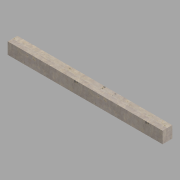
# Autodesk Inventor part: Bridge veneer
Saved by Autodesk Inventor 2022.1 (Build 261234020, 234B)
## iProperties
Created: 2021-10-21
Part Number: Bridge veneer
Material: Limestone
Document SubType Name: Modeling
Designer: awelt
Density: 2.6 g/cm^3
Appearance: Kasota Gray
Mass: 22240.5 g
Surface Area: 4243.54 cm^2
Volume: 8554.05 cm^3
Author: awelt
Autodesk Inventor part; units mm, degrees
ref_plane "YZ Plane" through (0, 0, 0) normal (1, 0, 0) x (0, 1, 0)
ref_plane "XZ Plane" through (0, 0, 0) normal (0, 1, 0) x (-1, 0, 0)
ref_plane "XY Plane" through (0, 0, 0) normal (0, 0, 1) x (1, 0, 0)
sketch "Sketch1" plane through (0, 0, 0) normal (0, 1, 0) x (-1, 0, 0)
  line L0 (609.6, -38.1) -> (-609.6, -38.1)
  line L1 (-609.6, -38.1) -> (-609.6, 38.1)
  line L2 (-609.6, 38.1) -> (609.6, 38.1)
  line L3 (609.6, 38.1) -> (609.6, -38.1)
  line L4 (609.6, -38.1) -> (-609.6, 38.1) construction
  line L5 (-609.6, -38.1) -> (609.6, 38.1) construction
  point P0 (0, 0)
  dimension "d0" = 1219.2
  dimension "d1" = 76.2
  constraints: 12 end point, 2 midpoint, 2 parallel, 1 horizontal, 1 perpendicular
  measures "d0" distance of L1.end L2.end
  measures "d1" distance of L0.end L1.end
extrude "Extrusion1" add sketch "Sketch1" along normal blind 92.075
sketch "Sketch2" plane through (609.6, 0, 38.1) normal (1, 0, 0) x (0, 0, -1)
  line L0 (0, 0) -> (0, 92.075) projected
  line L1 (0, 92.075) -> (76.2, 92.075) construction
  line L2 (0, 92.075) -> (0, 0) construction
  line L3 (0, 82.0217) -> (6.35, 82.0217)
  line L4 (6.35, 82.0217) -> (6.35, 75.6717)
  line L5 (6.35, 75.6717) -> (0, 75.6717)
  line L6 (0, 75.6717) -> (0, 82.0217) construction
  line L7 (0, 82.0217) -> (0, 75.6717)
  line L8 (0, 65.6184) -> (6.35, 65.6184)
  line L9 (6.35, 65.6184) -> (6.35, 59.2684)
  line L10 (6.35, 59.2684) -> (0, 59.2684)
  line L11 (0, 59.2684) -> (0, 65.6184)
  line L12 (0, 49.215) -> (6.35, 49.215)
  line L13 (6.35, 49.215) -> (6.35, 42.865)
  line L14 (6.35, 42.865) -> (0, 42.865)
  line L15 (0, 42.865) -> (0, 49.215)
  line L16 (0, 32.8117) -> (6.35, 32.8117)
  line L17 (6.35, 32.8117) -> (6.35, 26.4617)
  line L18 (6.35, 26.4617) -> (0, 26.4617)
  line L19 (0, 26.4617) -> (0, 32.8117)
  line L20 (0, 16.4084) -> (6.35, 16.4084)
  line L21 (6.35, 16.4084) -> (6.35, 10.0584)
  line L22 (6.35, 10.0584) -> (0, 10.0584)
  line L23 (0, 10.0584) -> (0, 16.4084)
  point P0 (38.1, 0)
  point P1 (0, 16.4084)
  point P2 (0, 10.0584)
  point P3 (0, 32.8117)
  point P4 (0, 26.4617)
  point P5 (0, 49.215)
  point P6 (0, 65.6184)
  point P7 (0, 59.2684)
  point P8 (0, 82.0217)
  point P9 (0, 75.6717)
  dimension "d5" = 6.35
  dimension "d6" = 6.35
  dimension "d7" = 6.35
  dimension "d8" = 6.35
  dimension "d9" = 10.0533
  dimension "d10" = 6.35
  dimension "d11" = 6.35
  dimension "d12" = 10.0533
  dimension "d13" = 10.0533
  dimension "d14" = 6.35
  dimension "d15" = 6.35
  dimension "d16" = 6.35
  dimension "d17" = 6.35
  dimension "d18" = 10.0533
  dimension "d19" = 10.0533
  dimension "d20" = 10.0584
  constraints: 44 end point, 10 parallel, 5 horizontal, 5 perpendicular, 5 point on line, 1 collinear, 1 vertical
  measures "d5" distance of L4.end L5.end
  measures "d6" distance of L3.end L4.end
  measures "d7" distance of L9.end L10.end
  measures "d8" distance of L8.end L9.end
  measures "d9" distance of L8.start L5.end
  measures "d10" distance of L13.end L14.end
  measures "d11" distance of L12.end L13.end
  measures "d12" distance of L12.start L10.end
  measures "d13" distance of L16.start L14.end
  measures "d14" distance of L16.end L17.end
  measures "d15" distance of L16.start L16.end
  measures "d16" distance of L21.end L22.end
  measures "d17" distance of L20.end L21.end
  measures "d18" distance of L20.start L18.end
  measures "d19" distance of L0.end L3.start
  measures "d20" distance of L0.start L22.end
extrude "Extrusion2" [suppressed]
equation "\"d12\" = d9"
equation "\"d13\" = d9"
equation "\"d18\" = d13"
